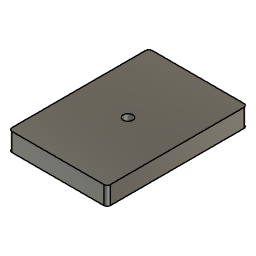
schlitten v2 (Autodesk Fusion 360 design; units mm, degrees)
Autodesk Fusion 360 part; units mm, degrees
sketch "Skizze1" plane through (0, 0, 0) normal (0, 0, 1) x (1, 0, 0)
  line L0 (0, 0) -> (88, 0)
  line L1 (88, 0) -> (88, 127)
  line L2 (88, 127) -> (0, 127)
  line L3 (0, 127) -> (0, 0)
  line L4 (-2, -2) -> (90, -2)
  line L5 (90, -2) -> (90, 129)
  line L6 (90, 129) -> (-2, 129)
  line L7 (-2, 129) -> (-2, -2)
  line L8 (2, 2) -> (86, 2)
  line L9 (86, 2) -> (86, 125)
  line L10 (86, 125) -> (2, 125)
  line L11 (2, 125) -> (2, 2)
  line L12 (86, 125) -> (2, 2) construction
  line L13 (2, 125) -> (86, 2) construction
  line L14 (34, 53.5) -> (54, 53.5)
  line L15 (54, 53.5) -> (54, 73.5)
  line L16 (54, 73.5) -> (34, 73.5)
  line L17 (34, 73.5) -> (34, 53.5)
  line L18 (34, 53.5) -> (54, 73.5) construction
  line L19 (54, 53.5) -> (34, 73.5) construction
  circle A0 centre (72.4, 63.5) radius 2.6
  line L20 (44, 2) -> (44, 125) construction
  circle A1 centre (72.4, 63.5) radius 5
  circle A2 centre (15.6, 63.5) radius 2.6
  circle A3 centre (15.6, 63.5) radius 5
  point P0 (44, 63.5)
  dimension "d1" = 88
  dimension "d2" = 127
  dimension "d3" = 2
  dimension "d4" = -2
  dimension "d15" = 20
  dimension "d16" = 20
  dimension "d21" = 5.2
  dimension "d22" = 13.6
  dimension "d23" = 10
  constraint horizontal L0
  constraint vertical L1
  constraint horizontal L2
  constraint vertical L3
  constraint coincident L0.start L3.end
  constraint horizontal L14
  constraint perpendicular L14 L15
  constraint parallel L14 L16
  constraint parallel L15 L17
  constraint coincident L18 P0
  constraint coincident L19 P0
  constraint midpoint L13 P0
  constraint midpoint L8 L20.start
  constraint midpoint L10 L20.end
  constraint concentric A0 A1
  constraint symmetric A0 L20 A2
  constraint symmetric L20 A1 A3
  measures "d1" distance of L0.start L0.end
  measures "d2" distance of L0.start L2.end
  measures "d15" distance of L15.end L16.end
  measures "d16" distance of L14.end L15.end
  measures "d21" diameter of A0
  measures "d22" distance of L9 A0.centre
  measures "d23" diameter of A1
extrude "Extrusion1" add sketch "Skizze1" along normal blind 2 contours L0 L1 L2 L3 | L4 L5 L6 L7 | L8 L9 L10 L11 | L14 L15 L16 L17 | A0 | A1 | A2 | A3
extrude "Extrusion2" add sketch "Skizze1" against normal blind 18.2 contours L0 L1 L2 L3
extrude "Extrusion3" add sketch "Skizze1" against normal blind 15 contours L4 L5 L6 L7
sketch "Skizze2" plane through (0, 0, -18.2) normal (0, 0, -1) x (1, 0, 0)
  line L0 (2, -125) -> (2, -2)
  line L1 (2, -2) -> (86, -2)
  line L2 (86, -2) -> (86, -125)
  line L3 (86, -125) -> (2, -125)
  line L4 (0, 0) -> (0, -127)
  line L5 (0, -127) -> (88, -127)
  line L6 (88, -127) -> (88, 0)
  line L7 (88, 0) -> (0, 0)
extrude "Extrusion4" cut sketch "Skizze2" against normal blind 6.4
fillet "Abrundung1" radius 3 4 edges at (90, -2, -6.5) (90, 129, -6.5) (-2, -2, -6.5) (-2, 129, -6.5)
sketch "Skizze3" plane through (0, 0, 0) normal (0, 0, 1) x (1, 0, 0)
  arc A0 (1, 129) -> (-2, 126) centre (1, 126) ccw construction
  line L0 (-2, 1) -> (-2, 126) construction
  line L1 (1, 129) -> (87, 129) construction
  arc A1 (90, 126) -> (87, 129) centre (87, 126) ccw construction
  line L2 (90, 126) -> (90, 1) construction
  arc A2 (87, -2) -> (90, 1) centre (87, 1) ccw construction
  line L3 (87, -2) -> (1, -2) construction
  arc A3 (-2, 1) -> (1, -2) centre (1, 1) ccw construction
extrude "Extrusion5" add sketch "Skizze1" against normal blind 11.8 contours L14 L15 L16 L17
fillet "Abrundung2" radius 2.5 4 edges at (34, 53.5, -5.9) (34, 73.5, -5.9) (54, 53.5, -5.9) (54, 73.5, -5.9)
extrude "Extrusion6" add sketch "Skizze1" against normal blind 11.8 contours A1 | A3
hole "Bohrung1" at (44, 63.5, 0) direction (0, 0, -1) diameter 8.86 depth 17 tip angle 118
extrude "Extrusion7" cut 1 faces at (42.0563, 65.454, 0) along direction (0, 0, 1) blind 56
equation "d7 = -15 mm - 3.2 mm"
equation "d17 = -15 mm + 3.2 mm"
equation "d22 = 11 mm + ( 5.2 / 2 ) * 1 mm"
equation "d24 = -15 mm + 3.2 mm"
